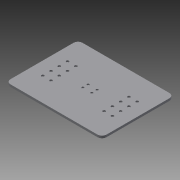
# Autodesk Inventor part: mic6_plate
Saved by Autodesk Inventor 2014 (Build 180170000, 170)
## iProperties
Created: 2014-08-09
Part Number: mic6_plate
Material: Generic
Document SubType Name: Modeling
Designer: Matthew
Density: 1 g/cm^3
Appearance: Default
Mass: 1147.76 g
Surface Area: 2727.3 cm^2
Volume: 1147.76 cm^3
Author: Matthew
Autodesk Inventor part; units mm, degrees
ref_plane "YZ Plane" through (0, 0, 0) normal (1, 0, 0) x (0, 1, 0)
ref_plane "XZ Plane" through (0, 0, 0) normal (0, 1, 0) x (-1, 0, 0)
ref_plane "XY Plane" through (0, 0, 0) normal (0, 0, 1) x (1, 0, 0)
sketch "Sketch1" plane through (0, 0, 0) normal (0, 1, 0) x (-1, 0, 0)
  line L0 (203.2, 152.4) -> (-203.2, 152.4)
  line L1 (-203.2, 152.4) -> (-203.2, -152.4)
  line L2 (-203.2, -152.4) -> (203.2, -152.4)
  line L3 (203.2, -152.4) -> (203.2, 152.4)
  line L4 (203.2, 152.4) -> (-203.2, -152.4) construction
  line L5 (-203.2, 152.4) -> (203.2, -152.4) construction
  point P0 (0, 0)
  dimension "d0" = 406.4
  dimension "d1" = 304.8
  constraints: 12 end point, 2 midpoint, 2 parallel, 1 horizontal, 1 perpendicular
  measures "d0" distance of L2.end L1.end
  measures "d1" distance of L0.end L1.end
extrude "Extrusion1" add sketch "Sketch1" along normal blind 9.525
fillet "Fillet1" radius 19.05 1 edges at (203.2, 4.7625, 152.4)
fillet "Fillet2" radius 19.05 1 edges at (203.2, 4.7625, -152.4)
fillet "Fillet3" radius 19.05 1 edges at (-203.2, 4.7625, 152.4)
fillet "Fillet4" radius 19.05 1 edges at (-203.2, 4.7625, -152.4)
sketch "Sketch2" plane through (0, 9.525, 0) normal (0, 1, 0) x (1, 0, 0)
  line L0 (-203.2, 152.4) -> (-203.2, -152.4) projected
  line L1 (-203.2, -152.4) -> (203.2, -152.4) projected
  point P0 (-203.2, 133.35)
  point P1 (-203.2, -133.35)
  point P2 (-184.15, -152.4)
  point P3 (184.15, -152.4)
  point P4 (0, 0)
  point P5 (-177.8, -127)
  point P6 (-177.8, -76.2)
  point P7 (-177.8, -25.4)
  point P8 (-177.8, 25.4)
  point P9 (-177.8, 76.2)
  point P10 (-177.8, 127)
  point P11 (-152.4, -127)
  point P12 (-152.4, -76.2)
  point P13 (-152.4, -25.4)
  point P14 (-152.4, 25.4)
  point P15 (-152.4, 76.2)
  point P16 (-152.4, 127)
  point P17 (-127, -127)
  point P18 (-127, -76.2)
  point P19 (-127, -25.4)
  point P20 (-127, 25.4)
  point P21 (-127, 76.2)
  point P22 (-127, 127)
  point P23 (-101.6, -127)
  point P24 (-101.6, -76.2)
  point P25 (-101.6, -25.4)
  point P26 (-101.6, 25.4)
  point P27 (-101.6, 76.2)
  point P28 (-101.6, 127)
  point P29 (-76.2, -127)
  point P30 (-76.2, -76.2)
  point P31 (-76.2, -25.4)
  point P32 (-76.2, 25.4)
  point P33 (-76.2, 76.2)
  point P34 (-76.2, 127)
  point P35 (-50.8, -127)
  point P36 (-50.8, -76.2)
  point P37 (-50.8, -25.4)
  point P38 (-50.8, 25.4)
  point P39 (-50.8, 76.2)
  point P40 (-50.8, 127)
  point P41 (-25.4, -127)
  point P42 (-25.4, -76.2)
  point P43 (-25.4, -25.4)
  point P44 (-25.4, 25.4)
  point P45 (-25.4, 76.2)
  point P46 (-25.4, 127)
  point P47 (0, -127)
  point P48 (0, -76.2)
  point P49 (0, -25.4)
  point P50 (0, 25.4)
  point P51 (0, 76.2)
  point P52 (0, 127)
  point P53 (25.4, -127)
  point P54 (25.4, -76.2)
  point P55 (25.4, -25.4)
  point P56 (25.4, 25.4)
  point P57 (25.4, 76.2)
  point P58 (25.4, 127)
  point P59 (50.8, -127)
  point P60 (50.8, -76.2)
  point P61 (50.8, -25.4)
  point P62 (50.8, 25.4)
  point P63 (50.8, 76.2)
  point P64 (50.8, 127)
  point P65 (76.2, -127)
  point P66 (76.2, -76.2)
  point P67 (76.2, -25.4)
  point P68 (76.2, 25.4)
  point P69 (76.2, 76.2)
  point P70 (76.2, 127)
  dimension "d8" = 25.4
  dimension "d9" = 25.4
  dimension "d12" = 50.8
  dimension "d15" = 25.4
  constraints: 1 horizontal, 1 vertical, 65 other
  measures "d8" distance from line of point (-177.8, -127) L1
  measures "d9" distance from line of L0 point (-177.8, -127)
  measures "d12" distance of point (-177.8, -127) point (-177.8, -76.2)
  measures "d15" distance of point (-177.8, -127) point (-152.4, -127)
hole "Hole1" at (-177.8, 9.525, 127) at (-177.8, 9.525, 76.2) at (-177.8, 9.525, 25.4) at (-177.8, 9.525, -25.4) at (-177.8, 9.525, -76.2) at (-177.8, 9.525, -127) at (-152.4, 9.525, 127) at (-152.4, 9.525, 76.2) at (-152.4, 9.525, 25.4) at (-152.4, 9.525, -25.4) at (-152.4, 9.525, -76.2) at (-152.4, 9.525, -127) at (-127, 9.525, 127) at (-127, 9.525, 76.2) at (-127, 9.525, 25.4) at (-127, 9.525, -25.4) at (-127, 9.525, -76.2) at (-127, 9.525, -127) at (-101.6, 9.525, 127) at (-101.6, 9.525, 76.2) at (-101.6, 9.525, 25.4) at (-101.6, 9.525, -25.4) at (-101.6, 9.525, -76.2) at (-101.6, 9.525, -127) at (-76.2, 9.525, 127) at (-76.2, 9.525, 76.2) at (-76.2, 9.525, 25.4) at (-76.2, 9.525, -25.4) at (-76.2, 9.525, -76.2) at (-76.2, 9.525, -127) at (-50.8, 9.525, 127) at (-50.8, 9.525, 76.2) at (-50.8, 9.525, 25.4) at (-50.8, 9.525, -25.4) at (-50.8, 9.525, -76.2) at (-50.8, 9.525, -127) at (-25.4, 9.525, 127) at (-25.4, 9.525, 76.2) at (-25.4, 9.525, 25.4) at (-25.4, 9.525, -25.4) at (-25.4, 9.525, -76.2) at (-25.4, 9.525, -127) at (0, 9.525, 127) at (0, 9.525, 76.2) at (0, 9.525, 25.4) at (0, 9.525, -25.4) at (0, 9.525, -76.2) at (0, 9.525, -127) at (25.4, 9.525, 127) at (25.4, 9.525, 76.2) direction (0, -1, 0) diameter 5.842 depth 25.4 tip angle 118 and at (25.4, 9.525, 25.4) (25.4, 9.525, -25.4) (25.4, 9.525, -76.2) (25.4, 9.525, -127) (50.8, 9.525, 127) (50.8, 9.525, 76.2) (50.8, 9.525, 25.4) (50.8, 9.525, -25.4) (50.8, 9.525, -76.2) (50.8, 9.525, -127) (76.2, 9.525, 127) (76.2, 9.525, 76.2) (76.2, 9.525, 25.4) (76.2, 9.525, -25.4) (76.2, 9.525, -76.2) (76.2, 9.525, -127)
sketch "Sketch3" plane through (0, 9.525, 0) normal (0, 1, 0) x (1, 0, 0)
  line L0 (-203.2, 152.4) -> (-203.2, -152.4) projected
  line L1 (203.2, 152.4) -> (-203.2, 152.4) projected
  line L2 (-153.9, 60) -> (-153.9, 10) construction
  line L3 (-153.9, 10) -> (-105.9, 10) construction
  line L4 (-105.9, 10) -> (-105.9, 60) construction
  line L5 (-105.9, 60) -> (-153.9, 60) construction
  line L6 (105.9, 60) -> (105.9, 10) construction
  line L7 (105.9, 10) -> (153.9, 10) construction
  line L8 (153.9, 10) -> (153.9, 60) construction
  line L9 (153.9, 60) -> (105.9, 60) construction
  line L10 (-153.9, -10) -> (-153.9, -60) construction
  line L11 (-153.9, -60) -> (-105.9, -60) construction
  line L12 (-105.9, -60) -> (-105.9, -10) construction
  line L13 (-105.9, -10) -> (-153.9, -10) construction
  line L14 (105.9, -10) -> (105.9, -60) construction
  line L15 (105.9, -60) -> (153.9, -60) construction
  line L16 (153.9, -60) -> (153.9, -10) construction
  line L17 (153.9, -10) -> (105.9, -10) construction
  line L18 (-24, 17.5) -> (24, 17.5) construction
  line L19 (24, 17.5) -> (24, -17.5) construction
  line L20 (24, -17.5) -> (-24, -17.5) construction
  line L21 (-24, -17.5) -> (-24, 17.5) construction
  line L22 (203.2, -152.4) -> (203.2, 152.4) projected
  point P0 (-184.15, 152.4)
  point P1 (-203.2, 133.35)
  point P2 (-203.2, -133.35)
  point P3 (184.15, 152.4)
  point P4 (0, 0)
  point P5 (-147.4, 52.5)
  point P6 (-112.4, 52.5)
  point P7 (-147.4, 17.5)
  point P8 (-112.4, 17.5)
  point P9 (112.4, 52.5)
  point P10 (147.4, 52.5)
  point P11 (112.4, 17.5)
  point P12 (147.4, 17.5)
  point P13 (-147.4, -17.5)
  point P14 (-112.4, -17.5)
  point P15 (-147.4, -52.5)
  point P16 (-112.4, -52.5)
  point P17 (112.4, -17.5)
  point P18 (147.4, -17.5)
  point P19 (112.4, -52.5)
  point P20 (147.4, -52.5)
  point P21 (0, 17.5)
  point P22 (129.9, 0)
  point P23 (24, 0)
  point P24 (129.9, 60)
  point P25 (-19, 11)
  point P26 (19, 11)
  point P27 (-19, -11)
  point P28 (19, -11)
  point P29 (203.2, -133.35)
  point P30 (203.2, 133.35)
  point P31 (-129.9, -60)
  dimension "d27" = 35
  dimension "d30" = 35
  dimension "d33" = 48
  dimension "d34" = 50
  dimension "d35" = 6.5
  dimension "d36" = 6.5
  dimension "d37" = 7.5
  dimension "d38" = 7.5
  dimension "d42" = 259.8
  dimension "d45" = 70
  dimension "d49" = 20
  dimension "d50" = 48
  dimension "d51" = 35
  dimension "d52" = 5
  dimension "d53" = 6.5
  dimension "d56" = 38
  dimension "d59" = 22
  dimension "d62" = 10
  dimension "d77" = 92.4
  dimension "d78" = 81.9
  dimension "d79" = 81.9
  dimension "d80" = 105.9
  dimension "d109" = 48
  dimension "d110" = 49.3
  dimension "d111" = 6.5
  dimension "d112" = 224.8
  constraints: 40 end point, 4 horizontal, 4 midpoint, 4 parallel, 3 perpendicular, 3 vertical, 2 horizontal alignment, 2 vertical alignment, 42 other
  measures "d27" distance of point (-147.4, 52.5) point (-112.4, 52.5)
  measures "d30" distance of point (-147.4, 52.5) point (-147.4, 17.5)
  measures "d33" distance of L2.end L3.end
  measures "d34" distance of L3.end L4.end
  measures "d35" distance from line of L4 point (-112.4, 52.5)
  measures "d36" distance from line of L2 point (-147.4, 52.5)
  measures "d37" distance from line of L5 point (-112.4, 52.5)
  measures "d38" distance from line of L3 point (-112.4, 17.5)
  measures "d42" distance of L2.start L6.start
  measures "d45" distance of L2.start L10.start
  measures "d49" distance between parallel lines of L3 L13
  measures "d50" distance of L19.end L20.end
  measures "d51" distance of L18.end L19.end
  measures "d52" distance from line of L21 point (-19, 11)
  measures "d53" distance from line of L18 point (-19, 11)
  measures "d56" distance of point (-19, 11) point (19, 11)
  measures "d59" distance of point (-19, 11) point (-19, -11)
  measures "d62" distance from line of L7 point (129.9, 0)
  measures "d77" distance between parallel lines of L1 L9
  measures "d78" distance between parallel lines of L21 L12
  measures "d79" distance between parallel lines of L14 L19
  measures "d80" horizontal distance of point (24, 0) point (129.9, 60)
  measures "d109" distance of L18.start L18.end
  measures "d110" distance between parallel lines of L22 L8
  measures "d111" distance from line of L6 point (112.4, 52.5)
  measures "d112" distance of point (112.4, -17.5) point (-112.4, -17.5)
hole "Hole4" at (-147.4, 9.525, -17.5) at (-147.4, 9.525, -52.5) at (-112.4, 9.525, -52.5) at (-112.4, 9.525, 17.5) at (-112.4, 9.525, -17.5) at (-147.4, 9.525, 17.5) at (-147.4, 9.525, 52.5) at (-112.4, 9.525, 52.5) at (112.4, 9.525, 17.5) at (147.4, 9.525, 17.5) at (147.4, 9.525, 52.5) at (112.4, 9.525, 52.5) at (112.4, 9.525, -52.5) at (147.4, 9.525, -17.5) at (112.4, 9.525, -17.5) at (147.4, 9.525, -52.5) direction (0, -1, 0) diameter 5 depth 25.4 tip angle 118
hole "Hole5" at (-19, 9.525, -11) at (19, 9.525, -11) at (-19, 9.525, 11) at (19, 9.525, 11) direction (0, -1, 0) diameter 4 depth 25.4 tip angle 118
hole "Hole6" at (-147.4, 9.525, -52.5) at (-112.4, 9.525, -52.5) at (-112.4, 9.525, -17.5) at (-147.4, 9.525, -17.5) at (-147.4, 9.525, 17.5) at (-112.4, 9.525, 17.5) at (-112.4, 9.525, 52.5) at (-147.4, 9.525, 52.5) at (112.4, 9.525, -52.5) at (147.4, 9.525, -52.5) at (147.4, 9.525, -17.5) at (112.4, 9.525, -17.5) at (112.4, 9.525, 17.5) at (147.4, 9.525, 17.5) at (147.4, 9.525, 52.5) at (112.4, 9.525, 52.5) direction (0, -1, 0) diameter 11.2 depth 6
hole "Hole7" at (-19, 9.525, -11) at (19, 9.525, -11) at (19, 9.525, 11) at (-19, 9.525, 11) direction (0, -1, 0) diameter 9.75 depth 5
equation "\"d62\" = 0.5 * d49"
equation "\"d79\" = d78"
body "Solid1"
